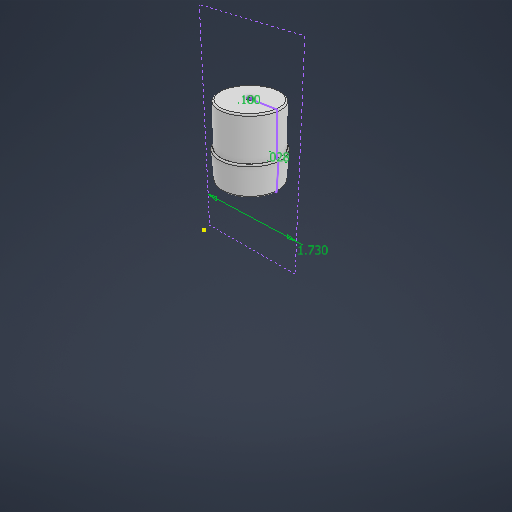
# Autodesk Inventor part: Part1
Saved by Autodesk Inventor 2025.2 (Build 292293000, 293)
## iProperties
Created: 2025-03-31
Part Number: Part1
Material: Generic
Document SubType Name: Modeling
Designer: mylap
Density: 1 g/cm^3
Appearance: Default
Author: mylap
Autodesk Inventor part; units mm, degrees
ref_plane "YZ Plane" through (0, 0, 0) normal (1, 0, 0) x (0, 1, 0)
ref_plane "XZ Plane" through (0, 0, 0) normal (0, 1, 0) x (-1, 0, 0)
ref_plane "XY Plane" through (0, 0, 0) normal (0, 0, 1) x (1, 0, 0)
sketch "Sketch1" plane through (0, 0, 0) normal (0, 0, 1) x (1, 0, 0)
  line L0 (3.6486, 85.3502) -> (47.5906, 85.3502) construction
  line L1 (47.5906, 85.3502) -> (47.5906, 3.7437) construction
  line L2 (47.5906, 3.7437) -> (3.6486, 3.7437) construction
  line L3 (3.6486, 3.7437) -> (3.6486, 85.3502) construction
  line L4 (38.1257, 32.1297) -> (38.7446, 44.3426)
  line L5 (38.0333, 44.3426) -> (37.7533, 60.8363)
  line L6 (25.8783, 44.547) -> (25.8783, 32.1297)
  line L7 (25.8783, 60.8363) -> (25.8783, 44.547)
  line L8 (38.1257, 32.1297) -> (25.8783, 32.1297)
  line L9 (37.7533, 60.8363) -> (25.8783, 60.8363)
  line L10 (38.7446, 44.3426) -> (25.8783, 44.3426)
  circle A0 centre (25.8783, 60.4685) radius 1.27
  point P0 (0, 0)
  point P1 (27.0939, 60.8363)
  point P2 (25.8783, 59.1985)
  dimension "d4" = 43.942
  dimension "d25" = 0.7112
  dimension "d37" = 2.54
  constraints: 14 end point, 3 horizontal, 3 point on line, 1 centre point, 1 perpendicular, 2 other
  measures "d4" distance between parallel lines of L1 L3
  measures "d25" distance from line of L4.end L5
  measures "d37" diameter of A0
revolve "Revolution2" add sketch "Sketch1" angle 360 about axis through (25.8783, 60.8363, 0) along (0, -1, 0) contours L8 L6 L10 L4 | L10 L6 L7 A0 L9 L5
fillet "Fillet1" radius 0.635 1 edges at (13.012, 44.3426, 0)
fillet "Fillet2" radius 0.635 1 edges at (13.631, 32.1297, 0)
fillet "Fillet3" radius 0.635 1 edges at (14.0033, 60.8363, 0)
body "Solid2"
